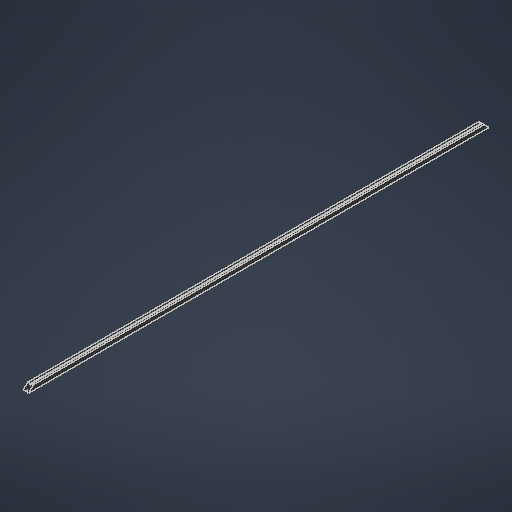
# Autodesk Inventor part: SP40-02 JUNTA INT 207
Saved by Autodesk Inventor 2025 (Build 290162000, 162)
## iProperties
Created: 2026-01-18
Part Number: SP40-02 JUNTA INT 207
Material: Caucho, negro
Document SubType Name: Modeling
Designer: ROLANDO
Density: 0.93 g/cm^3
Appearance: Caucho - Negro
Author: ROLANDO
Autodesk Inventor part; units mm, degrees
ref_plane "YZ Plane" through (0, 0, 0) normal (1, 0, 0) x (0, 1, 0)
ref_plane "XZ Plane" through (0, 0, 0) normal (0, 1, 0) x (-1, 0, 0)
sketch "Boceto1" plane through (0, 0, 0) normal (0, 0, 1) x (1, 0, 0)
  line L0 (28.5, 53.7) -> (28.5, 47.2)
  line L1 (26.1, 47.2) -> (28.5, 47.2)
  line L2 (26.1, 48.45) -> (25.3942, 48.45)
  line L3 (25.3942, 48.45) -> (24.7, 47.44)
  line L4 (26.1, 52.45) -> (25.3942, 52.45)
  line L5 (26.1, 53.7) -> (28.5, 53.7)
  line L6 (24.7, 53.46) -> (25.3942, 52.45)
  line L7 (26.1, 53.7) -> (26.1, 52.45)
  line L8 (26.1, 47.2) -> (26.1, 48.45)
  line L9 (21.2, 47.44) -> (24.7, 47.44)
  line L10 (21.2, 53.46) -> (21.2, 47.44)
  line L11 (21.2, 53.46) -> (24.7, 53.46)
  point P0 (28.5, 50.45)
  dimension "d78" = 6.5
  dimension "d88" = 2.4
  dimension "d95" = 6.02
  dimension "d100" = 2.4
  dimension "d108" = 4
  dimension "d109" = 0.7058
  dimension "d110" = 0.7058
  dimension "d145" = 2
  dimension "d146" = 2
  dimension "d150" = 3.5
  dimension "d151" = 3.5
  constraints: 24 end point, 3 horizontal, 3 vertical, 2 equal length, 1 midpoint
  measures "d78" distance between parallel lines of L1 L5
  measures "d88" distance between parallel lines of L0 L7
  measures "d95" distance of L3.end L6.start
  measures "d100" distance between parallel lines of L0 L8
  measures "d108" distance between parallel lines of L2 L4
  measures "d109" distance of L4.start L4.end
  measures "d110" distance of L2.start L2.end
  measures "d145" distance from line of point (28.5, 50.45) L4
  measures "d146" distance from line of point (28.5, 50.45) L2
  measures "d150" distance of L6.start L10.start
  measures "d151" distance of L9.start L9.end
extrude "Extrusión1" add sketch "Boceto1" against normal blind 617.8
ref_plane "Plano de trabajo1" through (0, 0, -308.9) normal (0, 0, 1) x (1, 0, 0)
sketch "Boceto2" plane through (28.5, -22.9, 0) normal (-1, 0, 0) x (0, 0, 1)
  line L0 (-617.8, 76.6) -> (-617.8, 70.1) projected
  line L1 (-617.8, 70.1) -> (-617.8, 76.6)
  line L2 (-617.8, 76.6) -> (-611.3, 76.6)
  line L3 (0, 76.6) -> (-617.8, 76.6) projected
  line L4 (-617.8, 70.1) -> (-611.3, 76.6)
  dimension "d149" = 45
  constraints: 6 end point, 1 point on line, 1 vertical
  measures "d149" angle of L0 L4
extrude "Extrusión2" cut sketch "Boceto2" along normal through all
mirror "Simetría1" about plane through (0, 0, -308.9) normal (0, 0, 1) of "Extrusión2"
